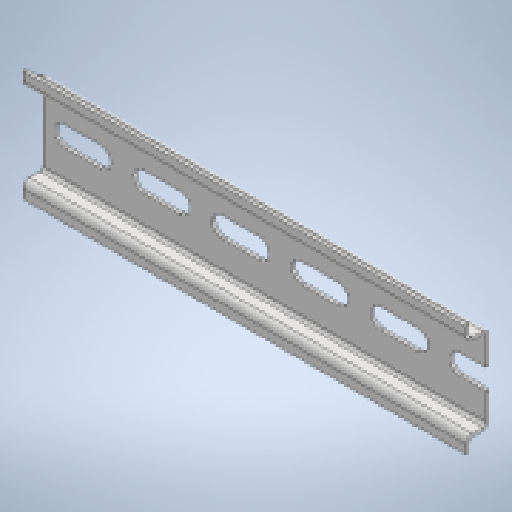
# Autodesk Inventor part: DIN-rail-short
Saved by Autodesk Inventor 2023 (Build 270158030, 158C)
## iProperties
Created: 2024-03-20
Part Number: DIN-rail-short
Material: Generic
Document SubType Name: Modeling
Designer: Imogen Heard
Density: 1 g/cm^3
Appearance: Default
Author: Imogen Heard
Autodesk Inventor part; units mm, degrees
ref_plane "YZ Plane" through (0, 0, 0) normal (1, 0, 0) x (0, 1, 0)
ref_plane "XZ Plane" through (0, 0, 0) normal (0, 1, 0) x (-1, 0, 0)
ref_plane "XY Plane" through (0, 0, 0) normal (0, 0, 1) x (1, 0, 0)
sketch "Sketch1" plane through (0, 0, 0) normal (1, 0, 0) x (0, 1, 0)
  line L0 (41.284, -14.8819) -> (64.684, -14.8819)
  line L1 (64.684, -13.8819) -> (41.284, -13.8819)
  line L2 (67.684, -8.5819) -> (70.484, -8.5819)
  line L3 (70.484, -8.5819) -> (70.484, -7.5819)
  line L4 (70.484, -7.5819) -> (67.684, -7.5819)
  line L5 (-1817770.1114, -20.3632) -> (-1817770.1114, -8.5819)
  line L6 (38.284, -7.5819) -> (35.484, -7.5819)
  line L7 (35.484, -7.5819) -> (35.484, -8.5819)
  line L8 (35.484, -8.5819) -> (38.284, -8.5819)
  line L9 (40.284, -9.5819) -> (40.284, -12.8819)
  arc A0 (67.684, -8.5819) -> (66.684, -9.5819) centre (67.684, -9.5819) ccw
  arc A1 (64.684, -13.8819) -> (65.684, -12.8819) centre (64.684, -12.8819) ccw
  arc A2 (40.284, -12.8819) -> (41.284, -13.8819) centre (41.284, -12.8819) ccw
  arc A3 (39.284, -9.5819) -> (38.284, -8.5819) centre (38.284, -9.5819) ccw
  arc A4 (40.284, -9.5819) -> (38.284, -7.5819) centre (38.284, -9.5819) ccw
  arc A5 (39.284, -12.8819) -> (41.284, -14.8819) centre (41.284, -12.8819) ccw
  line L10 (39.284, -9.5819) -> (39.284, -12.8819)
  arc A6 (67.684, -7.5819) -> (65.684, -9.5819) centre (67.684, -9.5819) ccw
  arc A7 (64.684, -14.8819) -> (66.684, -12.8819) centre (64.684, -12.8819) ccw
  line L11 (66.684, -9.5819) -> (66.684, -12.8819)
  line L12 (65.684, -9.5819) -> (65.684, -12.8819)
  line L13 (52.984, -4.8951) -> (52.984, -40.6352) construction
  line L14 (-285.558, -25.9225) -> (179.442, -25.9225) projected
  line L15 (179.442, -25.9225) -> (179.442, -22.9225) projected
  line L16 (-285.558, -22.9225) -> (179.442, -22.9225) projected
  line L17 (-285.558, -25.9225) -> (-285.558, -22.9225) projected
  point P0 (0, 0)
  point P1 (40.284, -11.2319)
  dimension "d0" = 1
  dimension "d1" = 1
  dimension "d5" = 35
  dimension "d8" = 7.3
  dimension "d9" = 1
  dimension "d10" = 1
  dimension "d11" = 2
  dimension "d12" = 2
  dimension "d13" = 12.7
  dimension "d15" = 12.7
  dimension "d16" = 4.8
  dimension "d17" = 4.8
  dimension "d20" = 1
  dimension "d21" = 1
  dimension "d22" = 2
  constraints: 28 end point, 17 point on circle, 12 tangent, 8 centre point, 7 horizontal alignment, 4 equal radius, 4 parallel, 3 perpendicular, 2 horizontal, 2 vertical, 1 midpoint, 1 point on line, 1 vertical alignment, 1 other
  measures "d0" distance between parallel lines of L2 L4
  measures "d1" distance between parallel lines of L0 L1
  measures "d5" distance between parallel lines of L7 L3
  measures "d8" distance between parallel lines of L4 L0
  measures "d9" radius of A0
  measures "d10" radius of A1
  measures "d11" radius of A4
  measures "d12" radius of A6
  measures "d13" distance between parallel lines of L13 L12
  measures "d15" distance between parallel lines of L13 L9
  measures "d16" distance between parallel lines of L9 L7
  measures "d17" distance between parallel lines of L12 L3
  measures "d20" distance between parallel lines of L12 L11
  measures "d21" distance between parallel lines of L10 L9
  measures "d22" radius of A5
extrude "Extrusion1" add sketch "Sketch1" along normal blind 300 contours A5 L10 A3 L8 L7 L6 A4 L9 A2 L1 A1 L12 A6 L4 L3 L2 A0 L11 A7 L0
sketch "Sketch2" plane through (0, 41.284, -13.8819) normal (0, 0, 1) x (1, 0, 0)
  line L0 (3.6, 11.7) -> (21.6, 11.7) construction
  line L1 (6.8, 8.5) -> (18.4, 8.5)
  line L2 (18.4, 14.9) -> (6.8, 14.9)
  arc A0 (6.8, 14.9) -> (6.8, 8.5) centre (6.8, 11.7) ccw
  arc A1 (18.4, 8.5) -> (18.4, 14.9) centre (18.4, 11.7) ccw
  line L3 (0, 29.2) -> (300, 29.2) projected
  line L4 (0, -5.8) -> (300, -5.8) projected
  line L5 (0, 23.4) -> (0, 0) projected
  arc A2 (31.8, 14.9) -> (31.8, 8.5) centre (31.8, 11.7) ccw
  line L6 (31.8, 8.5) -> (43.4, 8.5)
  arc A3 (43.4, 8.5) -> (43.4, 14.9) centre (43.4, 11.7) ccw
  line L7 (43.4, 14.9) -> (31.8, 14.9)
  arc A4 (56.8, 14.9) -> (56.8, 8.5) centre (56.8, 11.7) ccw
  line L8 (56.8, 8.5) -> (68.4, 8.5)
  arc A5 (68.4, 8.5) -> (68.4, 14.9) centre (68.4, 11.7) ccw
  line L9 (68.4, 14.9) -> (56.8, 14.9)
  arc A6 (81.8, 14.9) -> (81.8, 8.5) centre (81.8, 11.7) ccw
  line L10 (81.8, 8.5) -> (93.4, 8.5)
  arc A7 (93.4, 8.5) -> (93.4, 14.9) centre (93.4, 11.7) ccw
  line L11 (93.4, 14.9) -> (81.8, 14.9)
  arc A8 (106.8, 14.9) -> (106.8, 8.5) centre (106.8, 11.7) ccw
  line L12 (106.8, 8.5) -> (118.4, 8.5)
  arc A9 (118.4, 8.5) -> (118.4, 14.9) centre (118.4, 11.7) ccw
  line L13 (118.4, 14.9) -> (106.8, 14.9)
  arc A10 (131.8, 14.9) -> (131.8, 8.5) centre (131.8, 11.7) ccw
  line L14 (131.8, 8.5) -> (143.4, 8.5)
  arc A11 (143.4, 8.5) -> (143.4, 14.9) centre (143.4, 11.7) ccw
  line L15 (143.4, 14.9) -> (131.8, 14.9)
  arc A12 (156.8, 14.9) -> (156.8, 8.5) centre (156.8, 11.7) ccw
  line L16 (156.8, 8.5) -> (168.4, 8.5)
  arc A13 (168.4, 8.5) -> (168.4, 14.9) centre (168.4, 11.7) ccw
  line L17 (168.4, 14.9) -> (156.8, 14.9)
  arc A14 (181.8, 14.9) -> (181.8, 8.5) centre (181.8, 11.7) ccw
  line L18 (181.8, 8.5) -> (193.4, 8.5)
  arc A15 (193.4, 8.5) -> (193.4, 14.9) centre (193.4, 11.7) ccw
  line L19 (193.4, 14.9) -> (181.8, 14.9)
  line L20 (0, 0) -> (300, 0) projected
  line L21 (0, 24.4) -> (300, 24.4) projected
  line L22 (0, -1) -> (300, -1) projected
  arc A16 (206.8, 14.9) -> (206.8, 8.5) centre (206.8, 11.7) ccw
  line L23 (218.4, 14.9) -> (206.8, 14.9)
  arc A17 (218.4, 8.5) -> (218.4, 14.9) centre (218.4, 11.7) ccw
  line L24 (206.8, 8.5) -> (218.4, 8.5)
  arc A18 (231.8, 14.9) -> (231.8, 8.5) centre (231.8, 11.7) ccw
  line L25 (243.4, 14.9) -> (231.8, 14.9)
  arc A19 (243.4, 8.5) -> (243.4, 14.9) centre (243.4, 11.7) ccw
  line L26 (231.8, 8.5) -> (243.4, 8.5)
  arc A20 (256.8, 14.9) -> (256.8, 8.5) centre (256.8, 11.7) ccw
  line L27 (268.4, 14.9) -> (256.8, 14.9)
  arc A21 (268.4, 8.5) -> (268.4, 14.9) centre (268.4, 11.7) ccw
  line L28 (256.8, 8.5) -> (268.4, 8.5)
  arc A22 (281.8, 14.9) -> (281.8, 8.5) centre (281.8, 11.7) ccw
  line L29 (293.4, 14.9) -> (281.8, 14.9)
  arc A23 (293.4, 8.5) -> (293.4, 14.9) centre (293.4, 11.7) ccw
  line L30 (281.8, 8.5) -> (293.4, 8.5)
  point P0 (0, -41.284)
  point P1 (12.6, 11.7)
  point P2 (28.6, 11.7)
  point P3 (46.6, 11.7)
  point P4 (53.6, 11.7)
  point P5 (71.6, 11.7)
  point P6 (78.6, 11.7)
  point P7 (96.6, 11.7)
  point P8 (103.6, 11.7)
  point P9 (121.6, 11.7)
  point P10 (128.6, 11.7)
  point P11 (146.6, 11.7)
  point P12 (153.6, 11.7)
  point P13 (171.6, 11.7)
  point P14 (178.6, 11.7)
  point P15 (196.6, 11.7)
  point P16 (28.6, 11.7)
  point P17 (203.6, 11.7)
  point P18 (221.6, 11.7)
  point P19 (228.6, 11.7)
  point P20 (246.6, 11.7)
  point P21 (253.6, 11.7)
  point P22 (271.6, 11.7)
  point P23 (278.6, 11.7)
  point P24 (296.6, 11.7)
  dimension "d26" = 18
  dimension "d33" = 25
  dimension "d46" = 3.6
  dimension "d47" = 17.5
  dimension "d48" = 17.5
  dimension "d51" = 25
  constraints: 53 point on circle, 52 end point, 24 centre point, 4 tangent, 3 horizontal, 2 point on line, 1 midpoint, 1 parallel, 132 other
  measures "d26" distance of point (21.6, 11.7) point (3.6, 11.7)
  measures "d33" distance of A0.centre A2.centre
  measures "d46" distance from line of L5 point (3.6, 11.7)
  measures "d47" distance from line of L4 point (12.6, 11.7)
  measures "d48" distance from line of L3 point (12.6, 11.7)
  measures "d51" distance of point (178.6, 11.7) point (203.6, 11.7)
extrude "Extrusion2" cut sketch "Sketch2" against normal blind 25
sketch "Sketch3" plane through (0, 41.284, -13.8819) normal (0, 0, 1) x (1, 0, 0)
  line L0 (140, 34.2) -> (302, 34.2)
  line L1 (302, 34.2) -> (302, -10.8)
  line L2 (302, -10.8) -> (140, -10.8)
  line L3 (140, -10.8) -> (140, 34.2)
  line L4 (0, 23.4) -> (0, 0) projected
  line L5 (300, 23.4) -> (300, 0) projected
  line L6 (0, -5.8) -> (300, -5.8) projected
  line L7 (0, 29.2) -> (300, 29.2) projected
  point P0 (0, -41.284)
  dimension "d56" = 140
  dimension "d57" = 2
  dimension "d58" = 5
  dimension "d59" = 5
  constraints: 8 end point, 2 parallel, 1 horizontal, 1 perpendicular
  measures "d56" distance between parallel lines of L4 L3
  measures "d57" distance between parallel lines of L5 L1
  measures "d58" distance between parallel lines of L2 L6
  measures "d59" distance between parallel lines of L0 L7
extrude "Extrusion3" cut sketch "Sketch3" along normal through all both and the other way through all
equation "\"d39\" = d33"
